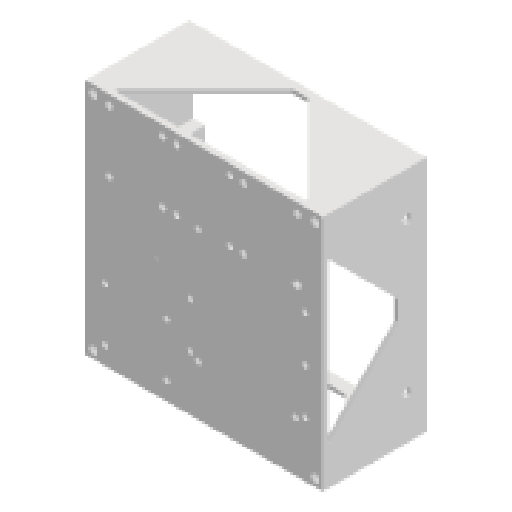
# Autodesk Inventor part: Bottom_carriage
Saved by Autodesk Inventor 2023 (Build 270158000, 158)
## iProperties
Created: 2021-02-01
Part Number: Bottom_carriage
Material: Generic
Document SubType Name: Modeling
Designer: CDT
Density: 1 g/cm^3
Appearance: Default
Author: CDT
Autodesk Inventor part; units mm, degrees
ref_plane "YZ Plane" through (0, 0, 0) normal (1, 0, 0) x (0, 1, 0)
ref_plane "XZ Plane" through (0, 0, 0) normal (0, 1, 0) x (-1, 0, 0)
ref_plane "XY Plane" through (0, 0, 0) normal (0, 0, 1) x (1, 0, 0)
sketch "Sketch1" plane through (0, 0, 0) normal (0, 0, 1) x (1, 0, 0)
  circle A0 centre (-66.09, 56.1166) radius 2
  circle A1 centre (45.91, 56.1166) radius 2
  circle A2 centre (45.91, -55.8834) radius 2
  circle A3 centre (-66.09, -55.8834) radius 2
  line L0 (49.91, -59.8834) -> (-70.09, -59.8834)
  line L1 (-70.09, -59.8834) -> (-70.09, 60.1166)
  line L2 (-70.09, 60.1166) -> (49.91, 60.1166)
  line L3 (49.91, 60.1166) -> (49.91, -59.8834)
  point P0 (0, 0)
  point P1 (-50.09, -79.8834)
  dimension "d11" = 4
  dimension "d12" = 4
  dimension "d13" = 4
  dimension "d14" = 4
  dimension "d150" = 4
  dimension "d151" = 4
  dimension "d152" = 4
  dimension "d153" = 4
  dimension "d154" = 4
  dimension "d155" = 4
  dimension "d156" = 4
  dimension "d157" = 4
  dimension "d158" = 120
  dimension "d159" = 120
  constraints: 8 end point, 4 centre point, 2 parallel, 1 horizontal, 1 perpendicular
  measures "d11" diameter of A0
  measures "d12" diameter of A1
  measures "d13" diameter of A2
  measures "d14" diameter of A3
  measures "d150" distance from line of L3 A2.centre
  measures "d151" distance from line of L0 A2.centre
  measures "d152" distance from line of L1 A3.centre
  measures "d153" distance from line of A3.centre L0
  measures "d154" distance from line of A0.centre L1
  measures "d155" distance from line of A0.centre L2
  measures "d156" distance from line of A1.centre L2
  measures "d157" distance from line of A1.centre L3
  measures "d158" distance of L1.end L2.end
  measures "d159" distance of L2.end L0.start
extrude "Extrusion1" add sketch "Sketch1" along normal blind 2
sketch "Sketch2" plane through (0, 0, 2) normal (0, 0, 1) x (1, 0, 0)
  line L0 (49.91, -59.8834) -> (49.91, -71.8834) projected
  line L1 (-70.09, 60.1166) -> (49.91, 60.1166)
  line L2 (49.91, 60.1166) -> (49.91, -59.8834)
  line L3 (49.91, -59.8834) -> (-70.09, -59.8834)
  line L4 (-70.09, -59.8834) -> (-70.09, 60.1166)
  circle A0 centre (-66.09, -55.8834) radius 2 projected
  circle A1 centre (-66.09, -55.8834) radius 2
  circle A2 centre (45.91, -55.8834) radius 2 projected
  circle A3 centre (45.91, -55.8834) radius 2
  circle A4 centre (45.91, 56.1166) radius 2 projected
  circle A5 centre (45.91, 56.1166) radius 2
  circle A6 centre (-66.09, 56.1166) radius 2 projected
  circle A7 centre (-66.09, 56.1166) radius 2
  constraints: 8 end point, 4 centre point, 4 coincident, 2 parallel, 1 horizontal, 1 perpendicular
extrude "Extrusion2" add sketch "Sketch2" along normal blind 0.5
sketch "Sketch8" plane through (0, 0, 0) normal (0, 0, -1) x (-1, 0, 0)
  circle A0 centre (-36.91, 24.1166) radius 1.75
  circle A1 centre (-36.91, 55.1166) radius 1.75
  circle A2 centre (-9.91, 24.1166) radius 1.75
  circle A3 centre (-9.91, 55.1166) radius 1.75
  line L0 (-49.91, -59.8834) -> (-49.91, 60.1166) projected
  line L1 (-49.91, 60.1166) -> (70.09, 60.1166) projected
  line L2 (70.09, -59.8834) -> (-49.91, -59.8834) projected
  point P0 (0, 0)
  point P1 (50.09, -79.8834)
  dimension "d88" = 3.5
  dimension "d89" = 3.5
  dimension "d90" = 3.5
  dimension "d91" = 3.5
  dimension "d92" = 31
  dimension "d93" = 27
  dimension "d94" = 27
  dimension "d95" = 31
  dimension "d96" = 13
  dimension "d97" = 13
  dimension "d98" = 31
  dimension "d99" = 5
  dimension "d108" = 84
  constraints: 4 centre point, 1 other
  measures "d88" diameter of A0
  measures "d89" diameter of A1
  measures "d90" diameter of A2
  measures "d91" diameter of A3
  measures "d92" distance of A1.centre A0.centre
  measures "d93" distance of A3.centre A1.centre
  measures "d94" distance of A2.centre A0.centre
  measures "d95" distance of A3.centre A2.centre
  measures "d96" distance from line of L0 A1.centre
  measures "d97" distance from line of L0 A0.centre
  measures "d98" vertical distance of A0.centre A3.centre
  measures "d99" distance from line of L1 A1.centre
extrude "Extrusion8" cut sketch "Sketch8" against normal blind 10
sketch "Sketch10" plane through (0, 0, 0) normal (0, 0, -1) x (-1, 0, 0)
  line L0 (70.09, -59.8834) -> (-49.91, -59.8834) projected
  line L1 (-49.91, 60.1166) -> (70.09, 60.1166) projected
  line L2 (-49.91, -59.8834) -> (70.09, -59.8834)
  line L3 (70.09, -59.8834) -> (70.09, 60.1166)
  line L4 (70.09, 60.1166) -> (-49.91, 60.1166)
  line L5 (-49.91, 60.1166) -> (-49.91, -59.8834)
  circle A0 centre (34.09, 0.1166) radius 0.5
  point P0 (0, 0)
  point P1 (-14.41, 60.1166)
  dimension "d127" = 120
  dimension "d128" = 120
  dimension "d129" = 1
  dimension "d130" = 60
  dimension "d131" = 84
  dimension "d166" = 36
  dimension "d167" = 60
  constraints: 8 end point, 2 parallel, 1 centre point, 1 horizontal, 1 perpendicular
  measures "d127" distance of L0.start L0.end
  measures "d128" distance of L2.end L1.end
  measures "d129" diameter of A0
  measures "d130" distance from line of A0.centre L0
  measures "d131" distance from line of A0.centre L5
  measures "d166" distance from line of L3 A0.centre
  measures "d167" distance from line of L1 A0.centre
extrude "Extrusion10" cut sketch "Sketch10" against normal blind 3 contours A0
pattern_linear "Rectangular Pattern4" count 3 spacing 34 along (-1, 0, 0) of "Extrusion8"
sketch "Sketch11" plane through (0, 0, 0) normal (0, 0, -1) x (-1, 0, 0)
  circle A0 centre (42.09, -17.3834) radius 1.475
  circle A1 centre (42.09, -17.3834) radius 3.35
  circle A2 centre (42.09, 17.6166) radius 1.475
  circle A3 centre (42.09, 17.6166) radius 3.35
  line L0 (70.09, 60.1166) -> (70.09, -59.8834) projected
  line L1 (-49.91, 60.1166) -> (70.09, 60.1166) projected
  line L2 (70.09, 60.1166) -> (-49.91, 60.1166)
  line L3 (-49.91, 60.1166) -> (-49.91, -59.8834)
  line L4 (-49.91, -59.8834) -> (70.09, -59.8834)
  line L5 (70.09, -59.8834) -> (70.09, 60.1166)
  circle A4 centre (34.09, 0.1166) radius 0.5 projected
  line L6 (42.09, 17.6166) -> (37.09, 17.6166)
  line L7 (37.09, 17.6166) -> (37.09, 21.0166)
  line L8 (37.09, 21.0166) -> (42.09, 21.0166)
  line L9 (42.09, 21.0166) -> (42.09, 17.6166)
  line L10 (42.09, 17.6166) -> (47.09, 17.6166)
  line L11 (47.09, 17.6166) -> (47.09, 21.0166)
  line L12 (47.09, 21.0166) -> (42.09, 21.0166)
  line L13 (42.09, 21.0166) -> (42.09, 17.6166)
  line L14 (42.09, -17.3834) -> (37.09, -17.3834)
  line L15 (37.09, -17.3834) -> (37.09, -20.7834)
  line L16 (37.09, -20.7834) -> (42.09, -20.7834)
  line L17 (42.09, -20.7834) -> (42.09, -17.3834)
  line L18 (42.09, -17.3834) -> (47.09, -17.3834)
  line L19 (47.09, -17.3834) -> (47.09, -20.7834)
  line L20 (47.09, -20.7834) -> (42.09, -20.7834)
  line L21 (42.09, -20.7834) -> (42.09, -17.3834)
  circle A5 centre (30.09, 17.6166) radius 1.5
  circle A6 centre (30.09, 17.6166) radius 3.5
  circle A7 centre (30.09, -17.3834) radius 1.5
  circle A8 centre (30.09, -17.3834) radius 3.5
  line L22 (30.09, -17.3834) -> (35.09, -17.3834)
  line L23 (35.09, -17.3834) -> (35.09, -20.7834)
  line L24 (35.09, -20.7834) -> (30.09, -20.7834)
  line L25 (30.09, -20.7834) -> (30.09, -17.3834)
  line L26 (30.09, -17.3834) -> (25.09, -17.3834)
  line L27 (25.09, -17.3834) -> (25.09, -20.7834)
  line L28 (25.09, -20.7834) -> (30.09, -20.7834)
  line L29 (30.09, -20.7834) -> (30.09, -17.3834)
  line L30 (30.09, 17.6166) -> (35.09, 17.6166)
  line L31 (35.09, 17.6166) -> (35.09, 21.0166)
  line L32 (35.09, 21.0166) -> (30.09, 21.0166)
  line L33 (30.09, 21.0166) -> (30.09, 17.6166)
  line L34 (30.09, 17.6166) -> (25.09, 17.6166)
  line L35 (25.09, 17.6166) -> (25.09, 21.0166)
  line L36 (25.09, 21.0166) -> (30.09, 21.0166)
  line L37 (30.09, 21.0166) -> (30.09, 17.6166)
  point P0 (0, 0)
  point P1 (50.09, -79.8834)
  point P2 (-14.41, 60.1166)
  point P3 (70.09, -59.8834)
  point P4 (38.74, 17.6166)
  point P5 (45.44, 17.6166)
  point P6 (45.44, -17.3834)
  point P7 (38.74, -17.3834)
  point P8 (26.44, 12.6166)
  point P9 (42.09, 20.9666)
  point P10 (19.74, 12.6166)
  point P11 (42.09, -20.7834)
  point P12 (26.44, -22.3834)
  point P13 (42.09, -20.7334)
  point P14 (19.74, -22.3834)
  point P15 (43.6666, 20.9166)
  point P16 (42.5134, 20.9166)
  point P17 (42.5134, -20.6834)
  point P18 (43.6666, -20.6834)
  point P19 (42.09, -20.7334)
  point P20 (42.09, 20.9666)
  point P21 (33.59, 17.6166)
  point P22 (26.59, 17.6166)
  point P23 (33.59, -17.3834)
  point P24 (26.59, -17.3834)
  dimension "d137" = 2.95
  dimension "d138" = 6.7
  dimension "d139" = 2.95
  dimension "d140" = 6.7
  dimension "d143" = 35
  dimension "d161" = 120
  dimension "d162" = 17.5
  dimension "d163" = 17.5
  dimension "d168" = 5
  dimension "d169" = 3.4
  dimension "d170" = 5
  dimension "d171" = 3.4
  dimension "d172" = 5
  dimension "d173" = 3.4
  dimension "d174" = 5
  dimension "d175" = 3.4
  dimension "d276" = 8
  dimension "d277" = 8
  dimension "d583" = 3
  dimension "d584" = 7
  dimension "d585" = 3
  dimension "d586" = 7
  dimension "d587" = 17.5
  dimension "d589" = 12
  dimension "d590" = 35
  dimension "d592" = 12
  dimension "d593" = 5
  dimension "d594" = 3.4
  dimension "d595" = 5
  dimension "d596" = 3.4
  dimension "d597" = 5
  dimension "d598" = 3.4
  dimension "d599" = 5
  dimension "d600" = 3.4
  constraints: 72 end point, 18 parallel, 9 horizontal, 9 perpendicular, 8 centre point, 4 coincident, 1 other
  measures "d137" diameter of A0
  measures "d138" diameter of A1
  measures "d139" diameter of A2
  measures "d140" diameter of A3
  measures "d143" distance of A0.centre A2.centre
  measures "d161" distance of L3.end L4.end
  measures "d162" vertical distance of A0.centre A4.centre
  measures "d163" vertical distance of A2.centre A4.centre
  measures "d168" distance of L7.end L8.end
  measures "d169" distance of L6.end L7.end
  measures "d170" distance of L12.end L11.end
  measures "d171" distance of L11.end L10.end
  measures "d172" distance of L16.end L15.end
  measures "d173" distance of L15.end L14.end
  measures "d174" distance of L19.end L20.end
  measures "d175" distance of L18.end L19.end
  measures "d276" horizontal distance of A2.centre A4.centre
  measures "d277" horizontal distance of A0.centre A4.centre
  measures "d583" diameter of A5
  measures "d584" diameter of A6
  measures "d585" diameter of A7
  measures "d586" diameter of A8
  measures "d587" vertical distance of A7.centre A4.centre
  measures "d589" distance of A0.centre L22.start
  measures "d590" distance of L30.start L22.start
  measures "d592" distance of A2.centre L30.start
  measures "d593" distance of L23.end L24.end
  measures "d594" distance of L22.end L23.end
  measures "d595" distance of L28.end L27.end
  measures "d596" distance of L27.end L26.end
  measures "d597" distance of L32.end L31.end
  measures "d598" distance of L31.end L30.end
  measures "d599" distance of L35.end L36.end
  measures "d600" distance of L34.end L35.end
extrude "Extrusion11" add sketch "Sketch11" along normal blind 20 contours L18 A1 L17 A0 | A0 L14 A1 L18 | A0 L17 A1 L14 | L18 L19 L20 L17 A1 | A1 L17 L16 L15 L14 | L10 A3 L6 A2 | A2 L9 A3 L10 | A2 L6 A3 L9 | A3 L9 L12 L11 L10 | A3 L6 L7 L8 L9 | L30 A6 L34 A5 | A5 L33 L32 A6 L30 | A5 L34 A6 L36 L33 | A6 L32 L31 L30 | L34 L35 L36 A6 | L22 A8 L24 L25 A7 | A7 L26 A8 L22 | A7 L25 L28 A8 L26 | L22 L23 L24 A8 | A8 L28 L27 L26
chamfer "Chamfer5" distance 0.65 angle 45 4 edges at (-45.44, 17.6166, -10) (-45.44, -17.3834, -10) (-38.74, -17.3834, -10) (-38.74, 17.6166, -10)
sketch "Sketch14" plane through (0, 0, 0) normal (0, 0, -1) x (-1, 0, 0)
  circle A0 centre (-40.91, -31.8834) radius 1.5
  circle A1 centre (-40.91, -8.8834) radius 1.5
  circle A2 centre (17.09, -31.8834) radius 1.5
  circle A3 centre (17.09, -8.8834) radius 1.5
  line L0 (70.09, 60.1166) -> (70.09, -59.8834) projected
  line L1 (-49.91, 60.1166) -> (70.09, 60.1166) projected
  circle A4 centre (-35.91, 23.6166) radius 1.5
  circle A5 centre (-35.91, -34.3834) radius 1.5
  circle A6 centre (13.09, 23.6166) radius 1.5
  circle A7 centre (13.09, -34.3834) radius 1.5
  line L2 (-49.91, -59.8834) -> (-49.91, 60.1166) projected
  line L3 (70.09, -59.8834) -> (-49.91, -59.8834) projected
  circle A8 centre (-40.91, 14.1166) radius 1.5
  point P0 (0, 0)
  point P1 (-14.41, 60.1166)
  dimension "d210" = 3
  dimension "d211" = 3
  dimension "d212" = 3
  dimension "d213" = 3
  dimension "d214" = 23
  dimension "d215" = 23
  dimension "d216" = 58
  dimension "d217" = 58
  dimension "d218" = 53
  dimension "d219" = 53
  dimension "d278" = 3
  dimension "d279" = 3
  dimension "d280" = 3
  dimension "d281" = 3
  dimension "d283" = 14
  dimension "d284" = 58
  dimension "d285" = 14
  dimension "d287" = 49
  dimension "d288" = 58
  dimension "d289" = 49
  dimension "d421" = 25.5
  dimension "d422" = 25.5
  dimension "d423" = 28
  dimension "d424" = 28
  dimension "d550" = 3
  dimension "d551" = 23
  dimension "d552" = 58
  constraints: 9 centre point
  measures "d210" diameter of A0
  measures "d211" diameter of A1
  measures "d212" diameter of A2
  measures "d213" diameter of A3
  measures "d214" distance of A1.centre A0.centre
  measures "d215" distance of A3.centre A2.centre
  measures "d216" distance of A0.centre A2.centre
  measures "d217" distance of A1.centre A3.centre
  measures "d218" distance from line of L0 A2.centre
  measures "d219" distance from line of L0 A3.centre
  measures "d278" diameter of A4
  measures "d279" diameter of A5
  measures "d280" diameter of A6
  measures "d281" diameter of A7
  measures "d283" distance from line of L2 A4.centre
  measures "d284" distance of A4.centre A5.centre
  measures "d285" distance from line of L2 A5.centre
  measures "d287" distance of A4.centre A6.centre
  measures "d288" distance of A7.centre A6.centre
  measures "d289" distance of A5.centre A7.centre
  measures "d421" distance from line of L3 A7.centre
  measures "d422" distance from line of L3 A5.centre
  measures "d423" distance from line of L3 A2.centre
  measures "d424" distance from line of L3 A0.centre
  measures "d550" diameter of A8
  measures "d551" distance of A1.centre A8.centre
  measures "d552" horizontal distance of A8.centre A3.centre
extrude "Extrusion14" cut sketch "Sketch14" against normal blind 10 contours A0 | A1 | A2 | A3 | A4 | A5 | A6 | A7 | A8
sketch "Sketch20" plane through (0, 0, 0) normal (0, 0, -1) x (-1, 0, 0)
  line L0 (70.09, 60.1166) -> (62.09, 60.1166)
  line L1 (62.09, 60.1166) -> (62.09, 52.1166)
  line L2 (62.09, 52.1166) -> (70.09, 52.1166)
  line L3 (70.09, 52.1166) -> (70.09, 60.1166)
  line L4 (-49.91, 60.1166) -> (70.09, 60.1166) projected
  line L5 (70.09, 60.1166) -> (70.09, -59.8834) projected
  circle A0 centre (66.09, 56.1166) radius 2 projected
  circle A1 centre (66.09, 56.1166) radius 2
  line L6 (70.09, 48.1166) -> (62.09, 48.1166)
  line L7 (62.09, 48.1166) -> (62.09, 40.1166)
  line L8 (62.09, 40.1166) -> (70.09, 40.1166)
  line L9 (70.09, 40.1166) -> (70.09, 48.1166)
  circle A2 centre (66.09, 44.1166) radius 2
  line L10 (-49.91, 60.1166) -> (-41.91, 60.1166)
  line L11 (-41.91, 60.1166) -> (-41.91, 53.1166)
  line L12 (-41.91, 53.1166) -> (-49.91, 53.1166)
  line L13 (-49.91, 53.1166) -> (-49.91, 60.1166)
  circle A3 centre (-45.91, 56.1166) radius 2 projected
  circle A4 centre (-45.91, 56.1166) radius 2
  line L14 (-49.91, 48.1166) -> (-41.91, 48.1166)
  line L15 (-41.91, 48.1166) -> (-41.91, 40.1166)
  line L16 (-41.91, 40.1166) -> (-49.91, 40.1166)
  line L17 (-49.91, 40.1166) -> (-49.91, 48.1166)
  line L18 (-49.91, -59.8834) -> (-49.91, 60.1166) projected
  line L19 (-41.91, 60.1166) -> (60.59, 60.1166) projected
  circle A5 centre (-45.91, 44.1166) radius 2
  line L20 (-41.91, 18.1166) -> (-49.91, 18.1166)
  line L21 (-49.91, 18.1166) -> (-49.91, 10.1166)
  line L22 (-49.91, 10.1166) -> (-41.91, 10.1166)
  line L23 (-41.91, 10.1166) -> (-41.91, 18.1166)
  line L24 (-41.91, -9.8834) -> (-49.91, -9.8834)
  line L25 (-49.91, -9.8834) -> (-49.91, -17.8834)
  line L26 (-49.91, -17.8834) -> (-41.91, -17.8834)
  line L27 (-41.91, -17.8834) -> (-41.91, -9.8834)
  line L28 (70.09, -59.8834) -> (-49.91, -59.8834) projected
  circle A6 centre (-45.91, 14.1166) radius 2
  circle A7 centre (-45.91, -13.8834) radius 2
  line L29 (-41.91, -51.8834) -> (-49.91, -51.8834)
  line L30 (-49.91, -51.8834) -> (-49.91, -59.8834)
  line L31 (-49.91, -59.8834) -> (-41.91, -59.8834)
  line L32 (-41.91, -59.8834) -> (-41.91, -51.8834)
  line L33 (-41.91, -39.8834) -> (-49.91, -39.8834)
  line L34 (-49.91, -39.8834) -> (-49.91, -47.8834)
  line L35 (-49.91, -47.8834) -> (-41.91, -47.8834)
  line L36 (-41.91, -47.8834) -> (-41.91, -39.8834)
  circle A8 centre (-45.91, -43.8834) radius 2
  circle A9 centre (-45.91, -55.8834) radius 2
  line L37 (70.09, -9.8834) -> (62.09, -9.8834)
  line L38 (62.09, -9.8834) -> (62.09, -17.8834)
  line L39 (62.09, -17.8834) -> (70.09, -17.8834)
  line L40 (70.09, -17.8834) -> (70.09, -9.8834)
  line L41 (70.09, -51.8834) -> (62.09, -51.8834)
  line L42 (62.09, -51.8834) -> (62.09, -59.8834)
  line L43 (62.09, -59.8834) -> (70.09, -59.8834)
  line L44 (70.09, -59.8834) -> (70.09, -51.8834)
  line L45 (70.09, -39.8834) -> (62.09, -39.8834)
  line L46 (62.09, -39.8834) -> (62.09, -47.8834)
  line L47 (62.09, -47.8834) -> (70.09, -47.8834)
  line L48 (70.09, -47.8834) -> (70.09, -39.8834)
  line L49 (62.09, 18.1166) -> (70.09, 18.1166)
  line L50 (70.09, 18.1166) -> (70.09, 10.1166)
  line L51 (70.09, 10.1166) -> (62.09, 10.1166)
  line L52 (62.09, 10.1166) -> (62.09, 18.1166)
  circle A10 centre (66.09, 14.1166) radius 2
  circle A11 centre (66.09, -13.8834) radius 2
  circle A12 centre (66.09, -43.8834) radius 2
  circle A13 centre (66.09, -55.8834) radius 2 projected
  circle A14 centre (66.09, -55.8834) radius 2
  point P0 (70.09, 48.1166)
  point P1 (-49.91, -9.8834)
  point P2 (-49.91, -17.8834)
  point P3 (-49.91, 18.1166)
  point P4 (-49.91, 10.1166)
  point P5 (-41.91, -59.8834)
  point P6 (-49.91, -51.8834)
  point P7 (-49.91, -39.8834)
  point P8 (70.09, -47.8834)
  point P9 (70.09, -39.8834)
  point P10 (70.09, -17.8834)
  point P11 (70.09, -9.8834)
  point P12 (70.09, 10.1166)
  point P13 (70.09, 18.1166)
  point P14 (62.09, -59.8834)
  point P15 (70.09, -51.8834)
  dimension "d303" = 8
  dimension "d304" = 8
  dimension "d305" = 0
  dimension "d306" = 0
  dimension "d307" = 4
  dimension "d308" = 4
  dimension "d309" = 8
  dimension "d310" = 8
  dimension "d311" = 12
  dimension "d312" = 0
  dimension "d313" = 4
  dimension "d314" = 4
  dimension "d315" = 4
  dimension "d317" = 7
  dimension "d326" = 8
  dimension "d327" = 8
  dimension "d328" = 0
  dimension "d329" = 12
  dimension "d330" = 4
  dimension "d331" = 4
  dimension "d332" = 4
  dimension "d333" = 8
  dimension "d334" = 8
  dimension "d335" = 8
  dimension "d336" = 8
  dimension "d337" = 42
  dimension "d338" = 42
  dimension "d339" = 0
  dimension "d340" = 0
  dimension "d341" = 4
  dimension "d342" = 4
  dimension "d343" = 4
  dimension "d344" = 4
  dimension "d345" = 4
  dimension "d346" = 4
  dimension "d347" = 8
  dimension "d348" = 8
  dimension "d349" = 0
  dimension "d350" = 0
  dimension "d351" = 8
  dimension "d352" = 8
  dimension "d353" = 0
  dimension "d354" = 12
  dimension "d355" = 4
  dimension "d356" = 4
  dimension "d357" = 4
  dimension "d359" = 4
  dimension "d360" = 4
  dimension "d361" = 4
  dimension "d362" = 4
  dimension "d363" = 8
  dimension "d364" = 8
  dimension "d365" = 8
  dimension "d366" = 8
  dimension "d367" = 8
  dimension "d368" = 8
  dimension "d369" = 8
  dimension "d370" = 8
  dimension "d371" = 0
  dimension "d372" = 0
  dimension "d373" = 42
  dimension "d374" = 42
  dimension "d375" = 12
  dimension "d376" = 0
  constraints: 96 end point, 24 parallel, 12 centre point, 12 horizontal, 12 perpendicular, 3 coincident
  measures "d303" distance of L2.end L1.end
  measures "d304" distance of L1.end L0.end
  measures "d305" distance between parallel lines of L4 L0
  measures "d306" distance between parallel lines of L5 L3
  measures "d307" distance from line of L5 A1.centre
  measures "d308" distance from line of L0 A1.centre
  measures "d309" distance of L8.end L7.end
  measures "d310" distance of L7.end L6.end
  measures "d311" distance between parallel lines of L4 L6
  measures "d312" distance between parallel lines of L5 L9
  measures "d313" diameter of A2
  measures "d314" distance from line of L9 A2.centre
  measures "d315" distance from line of L6 A2.centre
  measures "d317" distance of L10.end L11.end
  measures "d326" distance of L15.end L16.end
  measures "d327" distance of L14.end L15.end
  measures "d328" distance between parallel lines of L18 L17
  measures "d329" distance between parallel lines of L19 L14
  measures "d330" diameter of A5
  measures "d331" distance from line of L15 A5.centre
  measures "d332" distance from line of L14 A5.centre
  measures "d333" distance of L22.end L21.end
  measures "d334" distance of L21.end L20.end
  measures "d335" distance of L26.end L25.end
  measures "d336" distance of L25.end L24.end
  measures "d337" distance between parallel lines of L19 L20
  measures "d338" distance between parallel lines of L28 L26
  measures "d339" distance between parallel lines of L18 L21
  measures "d340" distance between parallel lines of L18 L25
  measures "d341" diameter of A6
  measures "d342" diameter of A7
  measures "d343" distance from line of L21 A6.centre
  measures "d344" distance from line of L20 A6.centre
  measures "d345" distance from line of L26 A7.centre
  measures "d346" distance from line of L25 A7.centre
  measures "d347" distance of L31.end L30.end
  measures "d348" distance of L30.end L29.end
  measures "d349" distance between parallel lines of L28 L31
  measures "d350" distance between parallel lines of L18 L30
  measures "d351" distance of L35.end L34.end
  measures "d352" distance of L34.end L33.end
  measures "d353" distance between parallel lines of L18 L34
  measures "d354" distance between parallel lines of L28 L35
  measures "d355" diameter of A8
  measures "d356" diameter of A9
  measures "d357" distance from line of L18 A8.centre
  measures "d359" distance from line of L36 A8.centre
  measures "d360" distance from line of L35 A8.centre
  measures "d361" distance from line of L18 A9.centre
  measures "d362" distance from line of L28 A9.centre
  measures "d363" distance of L39.end L38.end
  measures "d364" distance of L38.end L37.end
  measures "d365" distance of L43.end L42.end
  measures "d366" distance of L42.end L41.end
  measures "d367" distance of L47.end L46.end
  measures "d368" distance of L46.end L45.end
  measures "d369" distance of L50.end L51.end
  measures "d370" distance of L49.end L50.end
  measures "d371" distance between parallel lines of L28 L43
  measures "d372" distance between parallel lines of L5 L44
  measures "d373" distance between parallel lines of L28 L39
  measures "d374" distance between parallel lines of L19 L49
  measures "d375" distance between parallel lines of L28 L47
  measures "d376" distance between parallel lines of L5 L48
extrude "Extrusion18" add sketch "Sketch20" along normal blind 50 contours L3 L2 L1 L0 | L11 L12 L13 L4 | L5 L51 L52 L49 | L5 L39 L38 L37 | L20 L23 L22 L18 | L24 L27 L26 L18 | L5 L28 L42 L41 | L28 L18 L29 L32
sketch "Sketch21" plane through (0, 0, 0) normal (0, 0, -1) x (-1, 0, 0)
  line L0 (70.09, 60.1166) -> (70.09, -59.8834) projected
  line L1 (70.09, -59.8834) -> (-49.91, -59.8834) projected
  line L2 (70.09, 60.1166) -> (68.09, 60.1166)
  line L3 (68.09, 60.1166) -> (68.09, -59.8834)
  line L4 (68.09, -59.8834) -> (70.09, -59.8834)
  line L5 (70.09, -59.8834) -> (70.09, 60.1166)
  line L6 (-49.91, -59.8834) -> (-49.91, 60.1166) projected
  line L7 (70.09, -59.8834) -> (-49.91, -59.8834)
  line L8 (-49.91, -59.8834) -> (-49.91, -57.8834)
  line L9 (-49.91, -57.8834) -> (70.09, -57.8834)
  line L10 (70.09, -57.8834) -> (70.09, -59.8834)
  line L11 (-49.91, 60.1166) -> (70.09, 60.1166) projected
  line L12 (-49.91, -59.8834) -> (-47.91, -59.8834)
  line L13 (-47.91, -59.8834) -> (-47.91, 60.1166)
  line L14 (-47.91, 60.1166) -> (-49.91, 60.1166)
  line L15 (-49.91, 60.1166) -> (-49.91, -59.8834)
  line L16 (70.09, 60.1166) -> (-49.91, 60.1166)
  line L17 (-49.91, 60.1166) -> (-49.91, 58.1166)
  line L18 (-49.91, 58.1166) -> (70.09, 58.1166)
  line L19 (70.09, 58.1166) -> (70.09, 60.1166)
  line L20 (-41.91, 60.1166) -> (-49.91, 60.1166) projected
  line L21 (-49.91, 60.1166) -> (-41.91, 60.1166)
  line L22 (-41.91, 60.1166) -> (-41.91, 58.1166)
  line L23 (-41.91, 58.1166) -> (-49.91, 58.1166)
  line L24 (-49.91, 58.1166) -> (-49.91, 60.1166)
  point P0 (0, 0)
  point P1 (-47.91, -57.8834)
  point P2 (68.09, -57.8834)
  point P3 (70.09, -57.8834)
  point P4 (-47.91, 58.1166)
  point P5 (-41.91, 60.1166)
  point P6 (68.09, 58.1166)
  point P7 (-49.91, 60.1166)
  point P8 (-49.91, 60.1166)
  point P9 (-49.91, 60.1166)
  dimension "d388" = 2
  dimension "d389" = 2
  dimension "d390" = 2
  dimension "d393" = 120
  dimension "d394" = 2
  dimension "d395" = 8
  dimension "d396" = 2
  dimension "d516" = 120
  constraints: 40 end point, 10 parallel, 5 horizontal, 5 perpendicular, 3 point on line
  measures "d388" distance of L4.end L3.end
  measures "d389" distance of L7.end L8.end
  measures "d390" distance of L14.end L13.end
  measures "d393" distance of L18.end L17.end
  measures "d394" distance of L17.end L16.end
  measures "d395" distance of L22.end L23.end
  measures "d396" distance of L21.end L22.end
  measures "d516" distance of L0.end L1.end
extrude "Extrusion19" add sketch "Sketch21" along normal up to surface (50 mm away) contours L0 L18 L3 L2 | L0 L9 L3 L18 | L3 L18 L22 L11 | L22 L18 L13 L11 | L3 L1 L13 L9 | L13 L18 L6 L11 | L13 L1 L6 L9 | L9 L6 L18 L13
sketch "Sketch24" plane through (49.91, -59.8834, 2.5) normal (1, 0, 0) x (0, 0, -1)
  circle A0 centre (42.5, 98) radius 2
  line L0 (52.5, 120) -> (0, 120) projected
  circle A1 centre (42.5, 22) radius 2
  line L1 (52.5, 120) -> (52.5, 0) projected
  line L2 (52.5, 0) -> (0, 0) projected
  point P0 (2.5, 59.8834)
  point P1 (2.5, 120)
  point P2 (52.5, 118.5)
  dimension "d415" = 4
  dimension "d416" = 22
  dimension "d432" = 4
  dimension "d433" = 10
  dimension "d434" = 10
  dimension "d435" = 22
  constraints: 2 centre point
  measures "d415" diameter of A0
  measures "d416" distance from line of L0 A0.centre
  measures "d432" diameter of A1
  measures "d433" distance from line of L1 A1.centre
  measures "d434" distance from line of L1 A0.centre
  measures "d435" distance from line of L2 A1.centre
extrude "Extrusion22" cut sketch "Sketch24" against normal up to surface (120 mm away)
sketch "Sketch26" plane through (-70.09, 60.1166, 2.5) normal (0, 1, 0) x (1, 0, 0)
  line L0 (12, 48.5) -> (108, 48.5)
  line L1 (108, 48.5) -> (108, 3)
  line L2 (108, 3) -> (12, 3)
  line L3 (12, 3) -> (12, 48.5)
  line L4 (120, 52.5) -> (120, 0) projected
  line L5 (0, 0) -> (0, 52.5) projected
  line L6 (0, 52.5) -> (120, 52.5) projected
  line L7 (120, 0) -> (0, 0) projected
  point P0 (70.09, 2.5)
  dimension "d436" = 12
  dimension "d437" = 12
  dimension "d438" = 4
  dimension "d439" = 3
  constraints: 8 end point, 2 parallel, 1 horizontal, 1 perpendicular
  measures "d436" distance between parallel lines of L4 L1
  measures "d437" distance between parallel lines of L5 L3
  measures "d438" distance between parallel lines of L6 L0
  measures "d439" distance between parallel lines of L7 L2
extrude "Extrusion24" cut sketch "Sketch26" against normal blind 10 contours L0 L1 L2 L3
sketch "Sketch28" plane through (-70.09, -59.8834, 2.5) normal (0, -1, 0) x (1, 0, 0)
  line L0 (111, -46.5) -> (49, -46.5)
  line L1 (49, -46.5) -> (49, -2.5)
  line L2 (49, -2.5) -> (111, -2.5)
  line L3 (111, -2.5) -> (111, -46.5)
  line L4 (120, -52.5) -> (120, 0) projected
  line L5 (0, 0) -> (120, 0) projected
  dimension "d451" = 62
  dimension "d456" = 9
  dimension "d461" = 2.5
  dimension "d462" = 44
  constraints: 8 end point, 2 parallel, 1 horizontal, 1 perpendicular
  measures "d451" distance of L1.end L2.end
  measures "d456" distance between parallel lines of L4 L3
  measures "d461" distance between parallel lines of L5 L2
  measures "d462" distance between parallel lines of L0 L2
extrude "Extrusion26" cut sketch "Sketch28" against normal blind 10
chamfer "Chamfer10" distance 26 angle 45 2 edges at (-21.09, -58.8834, -44) (40.91, -58.8834, -44)
sketch "Sketch29" plane through (-70.09, -59.8834, 2.5) normal (0, -1, 0) x (1, 0, 0)
  line L0 (42, -2.5) -> (9, -2.5)
  line L1 (9, -2.5) -> (9, -47.5)
  line L2 (9, -47.5) -> (42, -47.5)
  line L3 (42, -47.5) -> (42, -2.5)
  line L4 (0, -52.5) -> (0, 0) projected
  line L5 (0, 0) -> (120, 0) projected
  line L6 (120, -52.5) -> (0, -52.5) projected
  point P0 (70.09, -2.5)
  dimension "d467" = 2.5
  dimension "d468" = 33
  dimension "d520" = 9
  dimension "d529" = 5
  constraints: 8 end point, 2 parallel, 1 horizontal, 1 perpendicular
  measures "d467" distance between parallel lines of L5 L0
  measures "d468" distance between parallel lines of L1 L3
  measures "d520" distance between parallel lines of L4 L1
  measures "d529" distance between parallel lines of L6 L2
extrude "Extrusion27" cut sketch "Sketch29" against normal blind 10
chamfer "Chamfer11" distance 15 angle 45 2 edges at (-61.09, -58.8834, -45) (-28.09, -58.8834, -45)
chamfer "Chamfer12" distance 44 angle 45 2 edges at (37.91, 59.1166, -46) (-58.09, 59.1166, -46)
sketch "Sketch32" plane through (41.91, -17.8834, 0) normal (-1, 0, 0) x (0, 0, 1)
  line L0 (-36, 0) -> (0, 0)
  line L1 (0, 0) -> (0, 36)
  line L2 (0, 36) -> (-36, 36)
  line L3 (-36, 36) -> (-36, 0)
  line L4 (0, 7.882) -> (0, 0) projected
  line L5 (0, 0) -> (-50, 0) projected
  line L6 (0, 36) -> (-50, 36) projected
  point P0 (0, 17.8834)
  point P1 (0, 8)
  dimension "d497" = 0
  dimension "d498" = 36
  dimension "d499" = 0
  dimension "d500" = 0
  constraints: 8 end point, 2 parallel, 1 horizontal, 1 perpendicular
  measures "d497" distance between parallel lines of L4 L1
  measures "d498" distance between parallel lines of L3 L1
  measures "d499" distance between parallel lines of L5 L0
  measures "d500" distance between parallel lines of L6 L2
extrude "Extrusion30" cut sketch "Sketch32" against normal up to surface (6 mm away)
sketch "Sketch33" plane through (49.91, -59.8834, 2.5) normal (1, 0, 0) x (0, 0, -1)
  line L0 (38.3, 100) -> (2.5, 100)
  line L1 (2.5, 100) -> (2.5, 20)
  line L2 (2.5, 20) -> (38.3, 20)
  line L3 (38.3, 20) -> (38.3, 100)
  line L4 (52.5, 0) -> (0, 0) projected
  line L5 (0, 0) -> (0, 120) projected
  line L6 (52.5, 120) -> (0, 120) projected
  point P0 (2.5, 59.8834)
  point P1 (2.5, 120)
  dimension "d506" = 35.8
  dimension "d508" = 20
  dimension "d509" = 2.5
  dimension "d530" = 20
  constraints: 8 end point, 2 parallel, 1 horizontal, 1 perpendicular
  measures "d506" distance of L2.end L1.end
  measures "d508" distance between parallel lines of L4 L2
  measures "d509" distance between parallel lines of L5 L1
  measures "d530" distance between parallel lines of L6 L0
extrude "Extrusion31" cut sketch "Sketch33" against normal up to surface (2 mm away)
chamfer "Chamfer16" distance 35 angle 45 2 edges at (48.91, -39.8834, -35.8) (48.91, 40.1166, -35.8)
chamfer "Chamfer17" distance 3 angle 45 2 edges at (-42.09, 14.2666, 0) (-42.09, -14.0334, 0)
sketch "Sketch34" plane through (-70.09, -59.8834, 2.5) normal (-1, 0, 0) x (0, 0, 1)
  circle A0 centre (-8, 106) radius 1.5
  circle A1 centre (-8, 57) radius 1.5
  line L0 (0, 120) -> (0, 0) projected
  line L1 (0, 120) -> (-52.5, 120) projected
  point P0 (-2.5, 59.8834)
  dimension "d521" = 3
  dimension "d522" = 3
  dimension "d523" = 8
  dimension "d524" = 8
  dimension "d525" = 49
  dimension "d526" = 14
  constraints: 2 centre point
  measures "d521" diameter of A0
  measures "d522" diameter of A1
  measures "d523" distance from line of L0 A0.centre
  measures "d524" distance from line of L0 A1.centre
  measures "d525" distance of A1.centre A0.centre
  measures "d526" distance from line of L1 A0.centre
extrude "Extrusion32" cut sketch "Sketch34" against normal blind 10
sketch "Sketch35" plane through (-62.09, 10.1166, 0) normal (1, 0, 0) x (0, 0, -1)
  line L0 (35, 8) -> (0, 8)
  line L1 (0, 8) -> (0, -28)
  line L2 (0, -28) -> (35, -28)
  line L3 (35, -28) -> (35, 8)
  line L4 (0, 8) -> (50, 8) projected
  line L5 (0, -28) -> (50, -28) projected
  line L6 (0, 8) -> (0, 42) projected
  point P0 (0, -10.1166)
  dimension "d531" = 0
  dimension "d532" = 0
  dimension "d533" = 0
  dimension "d534" = 35
  constraints: 8 end point, 2 parallel, 1 horizontal, 1 perpendicular
  measures "d531" distance between parallel lines of L4 L0
  measures "d532" distance between parallel lines of L5 L2
  measures "d533" distance between parallel lines of L6 L1
  measures "d534" distance between parallel lines of L1 L3
extrude "Extrusion33" cut sketch "Sketch35" against normal up to surface (6 mm away)
chamfer "Chamfer18" distance 6 angle 45 4 edges at (41.91, -13.8834, -36) (41.91, 14.1166, -36) (-62.09, 14.1166, -35) (-62.09, -13.8834, -35)
sketch "Sketch37" plane through (0, 0, 0) normal (0, 0, -1) x (-1, 0, 0)
  circle A0 centre (29.09, -23.7834) radius 1.5
  circle A1 centre (60.09, -23.7834) radius 1.5
  circle A2 centre (29.09, -50.7834) radius 1.5
  circle A3 centre (60.09, -50.7834) radius 1.5
  line L0 (37.09, -20.7834) -> (47.09, -20.7834) projected
  line L1 (68.09, 52.1166) -> (68.09, 18.1166) projected
  point P0 (0, 0)
  point P1 (68.09, -17.8834)
  point P2 (68.09, -51.8834)
  dimension "d556" = 3
  dimension "d557" = 3
  dimension "d558" = 3
  dimension "d559" = 3
  dimension "d560" = 3
  dimension "d561" = 31
  dimension "d562" = 3
  dimension "d564" = 8
  dimension "d565" = 8
  dimension "d566" = 31
  dimension "d567" = 27
  dimension "d568" = 27
  constraints: 4 centre point
  measures "d556" diameter of A0
  measures "d557" diameter of A1
  measures "d558" diameter of A2
  measures "d559" diameter of A3
  measures "d560" distance from line of L0 A0.centre
  measures "d561" distance of A0.centre A1.centre
  measures "d562" distance from line of L0 A1.centre
  measures "d564" distance from line of L1 A1.centre
  measures "d565" distance from line of L1 A3.centre
  measures "d566" distance of A2.centre A3.centre
  measures "d567" distance of A2.centre A0.centre
  measures "d568" distance of A1.centre A3.centre
extrude "Extrusion35" cut sketch "Sketch37" against normal blind 10
sketch "Sketch38" plane through (-70.09, -59.8834, 2.5) normal (-1, 0, 0) x (0, 0, 1)
  line L0 (-37, 20) -> (-2, 20)
  line L1 (-2, 20) -> (-2, 100)
  line L2 (-2, 100) -> (-37, 100)
  line L3 (-37, 100) -> (-37, 20)
  line L4 (0, 120) -> (0, 0) projected
  line L5 (-52.5, 0) -> (0, 0) projected
  line L6 (0, 120) -> (-52.5, 120) projected
  point P0 (-2.5, 59.8834)
  dimension "d571" = 35
  dimension "d572" = 2
  dimension "d573" = 20
  dimension "d574" = 20
  constraints: 8 end point, 2 parallel, 1 horizontal, 1 perpendicular
  measures "d571" distance between parallel lines of L3 L1
  measures "d572" distance between parallel lines of L4 L1
  measures "d573" distance between parallel lines of L5 L0
  measures "d574" distance between parallel lines of L6 L2
extrude "Extrusion36" cut sketch "Sketch38" against normal up to surface (2 mm away)
chamfer "Chamfer20" distance 35 angle 45 2 edges at (-69.09, 40.1166, -34.5) (-69.09, -39.8834, -34.5)
chamfer "Chamfer21" distance 1 angle 45 11 edges at (-68.09, -45.6334, 0) (-68.09, 45.8666, 0) (47.91, 46.6166, 0) (47.91, -45.8834, 0) (-24.59, -57.8834, 0) (41.41, -57.8834, 0) (-61.59, -57.8834, 0) (-61.09, -58.8834, 0) (40.91, -58.8834, 0) (-21.09, -58.8834, 0) (-28.09, -58.8834, 0)
chamfer "Chamfer22" distance 2 angle 45 8 edges at (-30.09, 14.1166, 0) (-30.09, -13.8834, 0) (-30.09, -20.7834, 0) (-35.09, -19.0834, 0) (-25.09, -19.0834, 0) (-25.09, 19.3166, 0) (-30.09, 21.0166, 0) (-35.09, 19.3166, 0)
equation "\"d13\" = d12"
equation "\"d14\" = d12"
equation "\"d97\" = d96"
equation "\"d98\" = d92"
equation "\"d138\" = d140"
body "Solid1"
